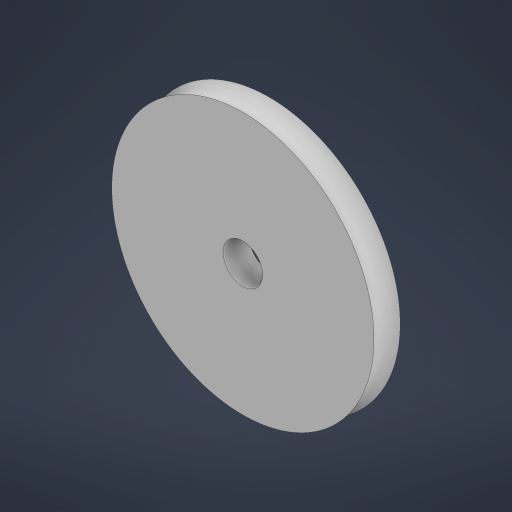
# Autodesk Inventor part: cable_roller
Saved by Autodesk Inventor 2024 (Build 280153000, 153)
## iProperties
Created: 2023-05-23
Part Number: cable_roller
Material: Generic
Document SubType Name: Modeling
Designer: aasmu
Density: 1 g/cm^3
Appearance: Default
cabel_roller_width: 4.000 mm
cabel_roller_OR: 20.000 mm
cabel_roller_IR: 3.000 mm
Author: aasmu
Autodesk Inventor part; units mm, degrees
ref_plane "YZ Plane" through (0, 0, 0) normal (1, 0, 0) x (0, 1, 0)
ref_plane "XZ Plane" through (0, 0, 0) normal (0, 1, 0) x (-1, 0, 0)
ref_plane "XY Plane" through (0, 0, 0) normal (0, 0, 1) x (1, 0, 0)
sketch "Sketch2" plane through (0, 0, 0) normal (0, 1, 0) x (-1, 0, 0)
  line L0 (20, 0) -> (0, 0)
  line L1 (0, 0) -> (0, -4) construction
  line L2 (0, -4) -> (20, -4)
  line L3 (20, -4) -> (20, 0) construction
  arc A0 (20, 0) -> (20, -4) centre (22, -2) ccw
  line L4 (3, 0) -> (3, -4)
  point P0 (20, -2)
  dimension "cabel_roller_width" = 4
  dimension "cabel_roller_OR" = 20
  dimension "cabel_roller_IR" = 3
  dimension "d4" = 90
  constraints: 10 end point, 3 perpendicular, 2 point on circle, 2 point on line, 1 centre point, 1 horizontal, 1 midpoint, 1 vertical
  measures "cabel_roller_width" distance of L0.end L1.end
  measures "cabel_roller_OR" distance of L1.end L2.end
  measures "cabel_roller_IR" distance from line of L1.end L4
revolve "Revolution1" add sketch "Sketch2" angle 360 about axis through (0, 0, 0) along (0, 0, -1)
equation "\"cabel_roller_OR\" = cabel_roller_OD"
equation "\"cabel_roller_IR\" = 0.5 * cabel_roller_ID"
equation "\"cabel_roller_OD\" = 20"
equation "\"cabel_roller_ID\" = 6"
body "Solid1"
